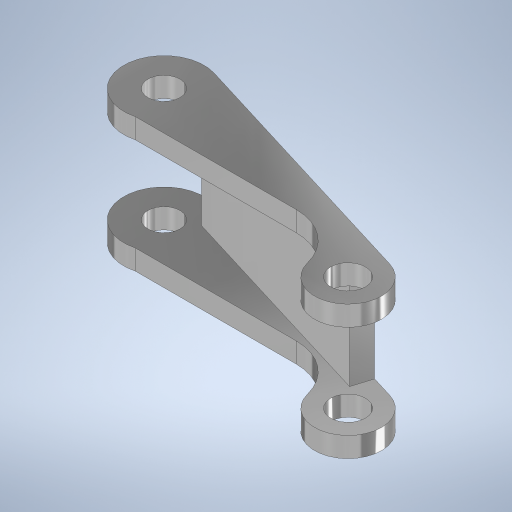
# Autodesk Inventor part: Lever for half overlay hinge
Saved by Autodesk Inventor 2024 (Build 280153000, 153)
## iProperties
Category: Perkama detale
Created: 2008-03-26
Part Number: Lever for half overlay hinge
Document SubType Name: Modeling
Designer: G.K.
Material: Steel
Description: Lever for half overlay hinge
Authority: Design by UAB Čeli APS
Mass: 3.43317 g
Surface Area: 7.77058 cm^2
Volume: 0.437347 cm^3
Density: 7.85 g/cm^3
Appearance: Chrome - Polished
Mase: 0.00343317
Author: Kestas
Autodesk Inventor part; units mm, degrees
ref_plane "YZ Plane" through (0, 0, 0) normal (1, 0, 0) x (0, 1, 0)
ref_plane "XZ Plane" through (0, 0, 0) normal (0, 1, 0) x (-1, 0, 0)
sketch "Sketch1" plane through (0, 0, 0) normal (0, 0, 1) x (1, 0, 0)
  circle A0 centre (17.6, 46.7) radius 1.2
  circle A1 centre (36.679, 41.3795) radius 1.3
  arc A2 (18.4785, 49.5685) -> (18.3735, 43.8014) centre (17.6, 46.7) ccw
  arc A3 (34.2538, 40.7726) -> (37.4111, 43.7699) centre (36.679, 41.3795) ccw
  line L0 (18.4785, 49.5685) -> (37.4111, 43.7699)
  line L1 (18.3735, 43.8014) -> (30.3735, 43.8014)
  arc A4 (34.2538, 40.7726) -> (30.3735, 43.8014) centre (30.3735, 39.8014) ccw
  circle A5 centre (36.679, 41.3795) radius 1.2
  point P0 (0, 0)
  dimension "d0" = 5
  dimension "d1" = 3
  dimension "d3" = 4
  dimension "d14" = 12
  dimension "d15" = 2.6
  constraints: 6 centre point, 6 point on circle, 5 end point, 4 tangent, 3 coincident, 1 horizontal, 4 other
  measures "d0" diameter of A3
  measures "d1" radius of A2
  measures "d3" radius of A4
  measures "d14" distance of L1.start L1.end
  measures "d15" diameter of A1
extrude "Extrusion1" add sketch "Sketch1" along normal mid plane 10 contours L0 A3 A4 L1 A2
ref_plane "Work Plane1" through (36.9719, 42.3357, 5) normal (0.2928471, 0.9561593, 0) x (0.9561593, -0.2928471, 0)
sketch "Sketch2" plane through (36.9719, 42.3357, 5) normal (0.2928471, 0.9561593, 0) x (0.9561593, -0.2928471, 0)
  line L0 (8.6668, 5) -> (-28.9168, 5) projected
  line L1 (-22.8007, 8.5) -> (2.5, 8.5)
  line L2 (2.5, 8.5) -> (2.5, 1.5)
  line L3 (2.5, 1.5) -> (-22.8007, 1.5)
  line L4 (-22.8007, 1.5) -> (-22.8007, 8.5)
  line L5 (2.5, 10) -> (2.5, 0) projected
  line L6 (-22.8007, 10) -> (-22.8007, 0) projected
  point P0 (-22.9531, 5)
  dimension "d7" = 7
  constraints: 8 end point, 2 collinear, 2 parallel, 1 horizontal, 1 perpendicular, 1 other
  measures "d7" distance of L3.end L1.start
extrude "Extrusion2" cut sketch "Sketch2" against normal through all
sketch "Sketch3" plane through (36.9719, 42.3357, 5) normal (-0.2928471, -0.9561593, 0) x (0.9561593, -0.2928471, 0)
  line L0 (-22.3987, -8.5) -> (-22.3987, -1.5) projected
  line L1 (-22.3987, -8.5) -> (2.2913, -8.5) projected
  line L2 (2.2913, -1.5) -> (2.2913, -8.5) projected
  line L3 (-22.3987, -1.5) -> (-18.3987, -1.5)
  line L4 (-18.3987, -1.5) -> (-18.3987, -8.5)
  line L5 (-18.3987, -8.5) -> (-22.3987, -8.5)
  line L6 (-22.3987, -8.5) -> (-22.3987, -1.5)
  line L7 (2.2913, -1.5) -> (-1.7087, -1.5)
  line L8 (-1.7087, -1.5) -> (-1.7087, -8.5)
  line L9 (-1.7087, -8.5) -> (2.2913, -8.5)
  line L10 (2.2913, -8.5) -> (2.2913, -1.5)
  point P0 (-22.9531, -5)
  dimension "d10" = 4
  dimension "d11" = 4
  constraints: 16 end point, 4 parallel, 2 horizontal, 2 perpendicular, 2 point on line
  measures "d10" distance between parallel lines of L4 L6
  measures "d11" distance between parallel lines of L2 L8
extrude "Extrusion3" cut sketch "Sketch3" against normal through all
body "Solid1"
